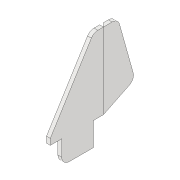
# Autodesk Inventor part: vertical_stablilizer
Saved by Autodesk Inventor 2019 (Build 230136000, 136)
## iProperties
Created: 2022-03-20
Part Number: vertical_stablilizer
Material: Foam board
Document SubType Name: Modeling
Designer: solyo
Density: 0.096049 g/cm^3
Appearance: Foam
Mass: 3.94114 g
Surface Area: 195.816 cm^2
Volume: 41.0326 cm^3
Author: solyo
Autodesk Inventor part; units mm, degrees
ref_plane "YZ Plane" through (0, 0, 0) normal (1, 0, 0) x (0, 1, 0)
ref_plane "XZ Plane" through (0, 0, 0) normal (0, 1, 0) x (-1, 0, 0)
ref_plane "XY Plane" through (0, 0, 0) normal (0, 0, 1) x (1, 0, 0)
sketch "Sketch1" plane through (0, 0, 0) normal (1, 0, 0) x (0, 1, 0)
  line L0 (0, 0) -> (-31, 0)
  line L1 (-31, 0) -> (-31, 42)
  line L2 (-31, 42) -> (0, 42)
  line L3 (0, 42) -> (0, 57)
  line L4 (0, 0) -> (0, -13)
  line L5 (0, -13) -> (20.1651, -54.3445)
  line L6 (100, -32) -> (100, 0)
  line L7 (100, 0) -> (8, 57)
  line L8 (20.1651, -54.3445) -> (100, -32)
  line L9 (8, 57) -> (0, 57)
  dimension "d0" = 31
  dimension "d1" = 42
  dimension "d2" = 15
  dimension "d3" = 13
  dimension "d4" = 46
  dimension "d5" = 154
  dimension "d6" = 100
  dimension "d8" = 32
  dimension "d14" = 8
  constraints: 20 end point, 3 perpendicular, 2 horizontal, 2 vertical, 1 horizontal alignment, 1 vertical alignment
  measures "d0" distance of L0.start L0.end
  measures "d1" distance of L0.end L1.end
  measures "d2" distance of L3.end L2.end
  measures "d3" distance of L0.start L4.end
  measures "d4" distance of L4.end L5.end
  measures "d5" angle of L5 L4
  measures "d6" distance between parallel lines of L6 L4
  measures "d8" distance of L6.start L6.end
  measures "d14" distance of L7.end L3.end
extrude "Extrusion1" add sketch "Sketch1" along normal mid plane 5
fillet "Fillet1" radius 10 4 edges at (0, 100, 0) (0, 100, -32) (0, -31, 42) (0, 20.1651, -54.3445)
sketch "Sketch2" plane through (-2.5, 0, -13) normal (0, -1, 0) x (1, 0, 0)
  line L0 (5, 0) -> (0, 0) projected
  line L1 (5, 13) -> (5, 0) projected
  line L2 (0, 13) -> (5, 13) projected
  line L3 (0, 0) -> (0, 13) projected
  line L4 (0, 0) -> (0, -5)
  line L5 (0, -41.3445) -> (0, 0) projected
  line L6 (5, 0) -> (0, -5)
  line L7 (5, 0) -> (0, 0) projected
  line L8 (5, 0) -> (0, 0)
  point P0 (2.5, 13)
  constraints: 6 end point, 1 collinear, 1 perpendicular, 1 point on line
extrude "Extrusion2" cut sketch "Sketch2" against normal through all contours L6 L4 L0
ref_plane "Work Plane1" through (-2.5, 0, -13) normal (0, 0, -1) x (-1, 0, 0)
split body "Split1" result two bodies by plane through (-2.5, 0, -13) normal (0, 0, -1) first body at (2, 42.7312, -26.0325)
equation "\"d9\" = Thickness"
equation "\"d12\" = Thickness"
equation "\"Thickness\" = 5"
